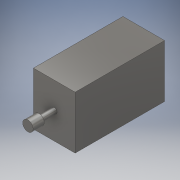
# Autodesk Inventor part: Solenoid
Saved by Autodesk Inventor 2019 (Build 230136000, 136)
## iProperties
Created: 2018-11-02
Part Number: Solenoid
Material: Generic
Document SubType Name: Modeling
Designer: Ethan
Density: 1 g/cm^3
Appearance: Semi-Polished
Author: Ethan
Autodesk Inventor part; units mm, degrees
ref_plane "YZ Plane" through (0, 0, 0) normal (1, 0, 0) x (0, 1, 0)
ref_plane "XZ Plane" through (0, 0, 0) normal (0, 1, 0) x (-1, 0, 0)
ref_plane "XY Plane" through (0, 0, 0) normal (0, 0, 1) x (1, 0, 0)
sketch "Sketch1" plane through (0, 0, 0) normal (0, 1, 0) x (-1, 0, 0)
  line L0 (-15, 32.2) -> (15, 32.2)
  line L1 (15, 32.2) -> (15, -32.2)
  line L2 (15, -32.2) -> (-15, -32.2)
  line L3 (-15, -32.2) -> (-15, 32.2)
  line L4 (-15, 32.2) -> (15, -32.2) construction
  line L5 (15, 32.2) -> (-15, -32.2) construction
  point P0 (0, 0)
  dimension "d0" = 30
  dimension "d1" = 64.4
  constraints: 12 end point, 2 midpoint, 2 parallel, 1 horizontal, 1 perpendicular
  measures "d0" distance of L1.end L2.end
  measures "d1" distance of L0.end L1.end
extrude "Extrusion1" add sketch "Sketch1" along normal mid plane 38
sketch "Sketch4" plane through (-15, 19, 32.2) normal (0, 0, 1) x (1, 0, 0)
  circle A0 centre (15, -19) radius 2
  dimension "d10" = 4
  constraints: 1 centre point, 1 coincident
  measures "d10" diameter of A0
extrude "Extrusion4" cut sketch "Sketch4" against normal through all
sketch "Sketch5" plane through (15, 19, -32.2) normal (0, 0, -1) x (-1, 0, 0)
  circle A0 centre (15, -19) radius 2 projected
  circle A1 centre (15, -19) radius 7.5
  point P0 (15, -19)
  dimension "d15" = 15
  constraints: 1 centre point, 1 coincident
  measures "d15" diameter of A1
extrude "Extrusion5" cut sketch "Sketch5" against normal blind 62.4
sketch "Sketch2" plane through (-15, 19, 32.2) normal (0, 0, 1) x (1, 0, 0)
  circle A0 centre (15, -19) radius 2
  dimension "d4" = 4
  constraints: 1 centre point, 1 coincident
  measures "d4" diameter of A0
extrude "Extrusion2" add sketch "Sketch2" along normal blind 11 and the other way blind 2 separate body
sketch "Sketch3" plane through (0, 0, 43.2) normal (0, 0, 1) x (1, 0, 0)
  circle A0 centre (0, 0) radius 3.75
  dimension "d7" = 7.5
  constraints: 1 centre point, 1 coincident
  measures "d7" diameter of A0
extrude "Extrusion3" add sketch "Sketch3" along normal blind 8 bodies 2
sketch "Sketch6" plane through (0, 0, 30.2) normal (0, 0, -1) x (-1, 0, 0)
  circle A0 centre (0, 0) radius 7.5
  dimension "d18" = 15
  constraints: 1 centre point, 1 coincident
  measures "d18" diameter of A0
extrude "Extrusion6" add sketch "Sketch6" along normal blind 68.4 bodies 2
sketch "Sketch7" plane through (15, 19, -32.2) normal (0, 0, -1) x (-1, 0, 0)
  circle A0 centre (15, -19) radius 3.75 projected
  circle A1 centre (15, -19) radius 12.5
  point P0 (15, -19)
  dimension "d21" = 25
  constraints: 1 centre point, 1 coincident
  measures "d21" diameter of A1
extrude "Extrusion7" add sketch "Sketch7" along normal blind 2 bodies 2
body "Solid1"
body "Solid2"
